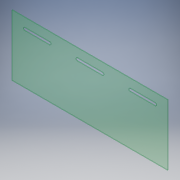
# Autodesk Inventor part: GBX_021.1-front-PMMA
Saved by Autodesk Inventor 2019 (Build 230136000, 136)
## iProperties
Created: 2019-09-28
Part Number: GBX_021.1-front-PMMA
Material: Generic
Document SubType Name: Modeling
Designer: Rene
Density: 1 g/cm^3
Appearance: Clear - Green 1
Author: Rene
Autodesk Inventor part; units mm, degrees
ref_plane "YZ Plane" through (0, 0, 0) normal (1, 0, 0) x (0, 1, 0)
ref_plane "XZ Plane" through (0, 0, 0) normal (0, 1, 0) x (-1, 0, 0)
ref_plane "XY Plane" through (0, 0, 0) normal (0, 0, 1) x (1, 0, 0)
sketch "Sketch1" plane through (0, 0, 0) normal (0, 0, 1) x (1, 0, 0)
  line L0 (350, -137.5) -> (-350, -137.5)
  line L1 (-350, -137.5) -> (-350, 137.5)
  line L2 (-350, 137.5) -> (350, 137.5)
  line L3 (350, 137.5) -> (350, -137.5)
  line L4 (350, -137.5) -> (-350, 137.5) construction
  line L5 (-350, -137.5) -> (350, 137.5) construction
  point P0 (0, 0)
  dimension "d0" = 275
  dimension "d1" = 700
  constraints: 12 end point, 2 midpoint, 2 parallel, 1 horizontal, 1 perpendicular
  measures "d0" distance of L0.end L1.end
  measures "d1" distance of L1.end L2.end
extrude "Extrusion1" add sketch "Sketch1" along normal blind 3
sketch "Sketch5" plane through (0, 0, 3) normal (0, 0, 1) x (1, 0, 0)
  line L0 (-300, 85.5) -> (-175, 85.5)
  line L1 (-175, 85.5) -> (-175, 97.5)
  line L2 (-175, 97.5) -> (-300, 97.5)
  line L3 (-300, 97.5) -> (-300, 85.5)
  line L4 (-62.5, 97.5) -> (62.5, 97.5)
  line L5 (62.5, 97.5) -> (62.5, 85.5)
  line L6 (62.5, 85.5) -> (-62.5, 85.5)
  line L7 (-62.5, 85.5) -> (-62.5, 97.5)
  line L8 (350, 137.5) -> (-350, 137.5) projected
  line L9 (175, 85.5) -> (300, 85.5)
  line L10 (300, 85.5) -> (300, 97.5)
  line L11 (300, 97.5) -> (175, 97.5)
  line L12 (175, 97.5) -> (175, 85.5)
  line L13 (-350, 137.5) -> (-350, -137.5) projected
  point P0 (0, 0)
  dimension "d21" = 12
  dimension "d29" = 40
  dimension "d30" = 40
  dimension "d33" = 40
  dimension "d35" = 50
  dimension "d36" = 50
  dimension "d37" = 112.5
  dimension "d38" = 112.5
  dimension "d41" = 12
  dimension "d42" = 12
  constraints: 24 end point, 6 parallel, 3 horizontal, 3 perpendicular
  measures "d21" distance between parallel lines of L2 L0
  measures "d29" distance between parallel lines of L8 L2
  measures "d30" distance between parallel lines of L8 L4
  measures "d33" distance between parallel lines of L8 L11
  measures "d35" distance between parallel lines of L13 L3
  measures "d36" horizontal distance of L8.start L10.end
  measures "d37" distance of L4.end L11.end
  measures "d38" distance of L1.end L4.start
  measures "d41" distance between parallel lines of L4 L6
  measures "d42" distance between parallel lines of L11 L9
extrude "Extrusion5" cut sketch "Sketch5" against normal blind 10
fillet "Fillet5" radius 6 4 edges at (-300, 97.5, 1.5) (-300, 85.5, 1.5) (-175, 85.5, 1.5) (-175, 97.5, 1.5)
fillet "Fillet6" radius 6 8 edges at (-62.5, 97.5, 1.5) (-62.5, 85.5, 1.5) (62.5, 97.5, 1.5) (62.5, 85.5, 1.5) (175, 97.5, 1.5) (175, 85.5, 1.5) (300, 97.5, 1.5) (300, 85.5, 1.5)
equation "\"d30\" = d29"
equation "\"d33\" = d29"
equation "\"d41\" = d21"
equation "\"d42\" = d21"
equation "\"d40\" = 0.5 * d21"
equation "\"d43\" = 0.5 * d21"
body "Solid1"
